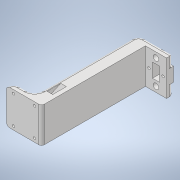
# Autodesk Inventor part: Joint_Tubes_1_2
Saved by Autodesk Inventor 2022.3 (Build 263350000, 350)
## iProperties
Created: 2023-03-29
Part Number: Joint_Tubes_1_2
Material: Generic
Document SubType Name: Modeling
Designer: Manuel Hueso Béjar
Density: 1 g/cm^3
Appearance: Default
Author: Manuel Hueso Béjar
Autodesk Inventor part; units mm, degrees
ref_plane "YZ Plane" through (0, 0, 0) normal (1, 0, 0) x (0, 1, 0)
ref_plane "XZ Plane" through (0, 0, 0) normal (0, 1, 0) x (-1, 0, 0)
ref_plane "XY Plane" through (0, 0, 0) normal (0, 0, 1) x (1, 0, 0)
sketch "Sketch1" plane through (0, 0, 0) normal (0, 1, 0) x (-1, 0, 0)
  line L0 (-10, 74) -> (10, 74)
  line L1 (10, 74) -> (10, -74)
  line L2 (10, -74) -> (-10, -74)
  line L3 (-10, -74) -> (-10, 74)
  line L4 (-10, 74) -> (10, -74) construction
  line L5 (10, 74) -> (-10, -74) construction
  line L6 (-10, 74) -> (40, 74)
  line L7 (40, 74) -> (40, 64)
  line L8 (40, 64) -> (-10, 64)
  line L9 (-10, 64) -> (-10, 74)
  line L10 (10, -74) -> (-40, -74)
  line L11 (-40, -74) -> (-40, -84)
  line L12 (-40, -84) -> (10, -84)
  line L13 (10, -84) -> (10, -74)
  point P0 (0, 0)
  point P1 (-10, -74)
  point P2 (10, 64)
  dimension "d0" = 20
  dimension "d1" = 148
  dimension "d2" = 50
  dimension "d3" = 10
  dimension "d4" = 50
  dimension "d5" = 10
  constraints: 28 end point, 6 parallel, 3 horizontal, 3 perpendicular, 2 midpoint
  measures "d0" distance of L1.end L2.end
  measures "d1" distance of L0.end L1.end
  measures "d2" distance of L7.end L8.end
  measures "d3" distance of L6.end L7.end
  measures "d4" distance of L12.end L11.end
  measures "d5" distance of L11.end L10.end
extrude "Extrusion1" add sketch "Sketch1" along normal blind 50
fillet "Fillet1" radius 10 2 edges at (-10, 25, -84) (-10, 25, 64)
fillet "Fillet2" radius 5 14 edges at (19.9999, 50, -84) (-10, 50, -9.9999) (-10, 50, -74) (-12.9289, 50, 61.0711) (-29.9999, 50, 64) (-7.0711, 50, -81.0711) (-10, 0, -74) (-7.0711, 0, -81.0711) (-10, 0, -9.9999) (-12.9289, 0, 61.0711) (-29.9999, 0, 64) (19.9999, 0, -84) (-40, 50, 69) (-40, 0, 69)
fillet "Fillet3" radius 10 3 edges at (-38.5355, 48.5355, 65.4645) (-38.5355, 1.4645, 65.4645) (-40, 25, 64)
sketch "Sketch2" plane through (10, 0, 74) normal (0, 0, 1) x (1, 0, 0)
  line L0 (0, 50) -> (-10, 50)
  line L1 (-10, 50) -> (-10, 45)
  line L2 (-10, 45) -> (0, 45)
  line L3 (0, 45) -> (0, 50)
  line L4 (-10, 0) -> (-10, 5) projected
  line L5 (0, 0) -> (-10, 0)
  line L6 (-10, 0) -> (-10, 5)
  line L7 (-10, 5) -> (0, 5)
  line L8 (0, 5) -> (0, 0)
  line L9 (0, 50) -> (-40, 50)
  line L10 (-40, 50) -> (-40, 45)
  line L11 (-40, 45) -> (0, 45)
  line L12 (0, 45) -> (0, 50)
  line L13 (0, 0) -> (-40, 0)
  line L14 (-40, 0) -> (-40, 5)
  line L15 (-40, 5) -> (0, 5)
  line L16 (0, 5) -> (0, 0)
  circle A0 centre (-10, 5) radius 1.7
  circle A1 centre (-10, 45) radius 1.7
  circle A2 centre (-40, 5) radius 1.7
  circle A3 centre (-40, 45) radius 1.7
  dimension "d11" = 10
  dimension "d12" = 5
  dimension "d13" = 10
  dimension "d14" = 5
  dimension "d15" = 40
  dimension "d16" = 5
  dimension "d17" = 40
  dimension "d18" = 5
  dimension "d19" = 3.4
  dimension "d20" = 3.4
  dimension "d21" = 3.4
  dimension "d22" = 3.4
  constraints: 32 end point, 8 parallel, 4 centre point, 4 coincident, 4 horizontal, 4 perpendicular
  measures "d11" distance of L2.end L1.end
  measures "d12" distance of L1.end L0.end
  measures "d13" distance of L4.end L7.end
  measures "d14" distance of L5.end L4.end
  measures "d15" distance of L11.end L10.end
  measures "d16" distance of L10.end L9.end
  measures "d17" distance of L14.end L15.end
  measures "d18" distance of L13.end L14.end
  measures "d19" diameter of A0
  measures "d20" diameter of A1
  measures "d21" diameter of A2
  measures "d22" diameter of A3
extrude "Extrusion2" cut sketch "Sketch2" against normal up to surface (10 mm away) contours A1 L2 L1 | L1 L11 A1 | A1 L11 L2 | A3 L11 L10 | L10 L11 A3 | A0 L15 L4 | L4 L7 A0 | L15 A0 L7 | A2 L15 L14 | L14 L15 A2
sketch "Sketch3" plane through (-20, 5, 64) normal (0, 0, -1) x (-1, 0, 0)
  circle A0 centre (10, 40) radius 1.7 projected
  arc A1 (10, 1.7) -> (8.3, 0) centre (10, 0) ccw projected
  line L0 (10, 40) -> (10, 0)
  point P0 (-20, -5)
  constraints: 2 end point, 1 vertical
hole "Hole1" at (-30, 45, 64) at (-30, 5, 64) direction (0, 0, 1) diameter 3.4 depth 2.2 countersink diameter 6 countersink angle 90
sketch "Sketch4" plane through (0, 45, 64) normal (0, 0, 1) x (1, 0, 0)
  line L0 (-4, -4) -> (4, -4)
  line L1 (4, -4) -> (4, 4)
  line L2 (4, 4) -> (-4, 4)
  line L3 (-4, 4) -> (-4, -4)
  line L4 (40, 0) -> (0, 0) projected
  line L5 (-4, -4) -> (4, 4) construction
  line L6 (4, -4) -> (-4, 4) construction
  point P0 (0, -45)
  dimension "d32" = 8
  dimension "d33" = 8
  constraints: 12 end point, 2 midpoint, 2 parallel, 1 horizontal, 1 perpendicular
  measures "d32" distance of L2.end L1.end
  measures "d33" distance of L1.end L0.end
sketch "Sketch5" plane through (10, 0, 74) normal (1, 0, 0) x (0, 0, -1)
  line L0 (0, 45) -> (20, 45)
  line L1 (20, 45) -> (20, 50)
  line L2 (20, 50) -> (0, 50)
  line L3 (0, 50) -> (0, 45)
  line L4 (20, 47.5) -> (40, 47.5)
  line L5 (40, 47.5) -> (40, 56.5)
  line L6 (40, 56.5) -> (20, 56.5)
  line L7 (20, 56.5) -> (20, 47.5)
  line L8 (20, 47.5) -> (40, 56.5)
  line L9 (0, 50) -> (148, 50) projected
  line L10 (0, 0) -> (0, 50) projected
  line L11 (20, 47.5) -> (10, 47.5)
  point P0 (74, 0)
  point P1 (148, 50)
  dimension "d34" = 20
  dimension "d35" = 5
  dimension "d36" = 20
  dimension "d37" = 9
  dimension "d38" = 0
  dimension "d39" = 0
  constraints: 20 end point, 4 parallel, 3 horizontal, 2 perpendicular, 1 midpoint, 1 other
  measures "d34" distance of L2.end L1.end
  measures "d35" distance of L1.end L0.end
  measures "d36" distance of L6.end L5.end
  measures "d37" distance of L5.end L4.end
  measures "d38" vertical extent of L2
  measures "d39" distance between parallel lines of L10 L3
sweep "Sweep1" cut profiles "Sketch4" path "Sketch5" path curves L11 L8
sketch "Sketch6" plane through (0, 5, 64) normal (0, 0, 1) x (1, 0, 0)
  line L0 (-4, -4) -> (4, -4)
  line L1 (4, -4) -> (4, 4)
  line L2 (4, 4) -> (-4, 4)
  line L3 (-4, 4) -> (-4, -4)
  line L4 (-10, 0) -> (0, 0) projected
  line L5 (-4, -4) -> (4, 4) construction
  line L6 (4, -4) -> (-4, 4) construction
  point P0 (0, -5)
  dimension "d42" = 8
  dimension "d43" = 8
  constraints: 12 end point, 2 midpoint, 2 parallel, 1 horizontal, 1 perpendicular
  measures "d42" distance of L2.end L1.end
  measures "d43" distance of L1.end L0.end
sketch "Sketch7" plane through (10, 0, 74) normal (1, 0, 0) x (0, 0, -1)
  line L0 (5, 0) -> (0, 0) projected
  line L1 (0, 0) -> (20, 0)
  line L2 (20, 0) -> (20, 5)
  line L3 (20, 5) -> (0, 5)
  line L4 (0, 5) -> (0, 0)
  line L5 (20, 2.5) -> (10, 2.5)
  line L6 (20, 2.5) -> (40, 2.5)
  line L7 (40, 2.5) -> (40, -6.5)
  line L8 (40, -6.5) -> (20, -6.5)
  line L9 (20, -6.5) -> (20, 2.5)
  line L10 (20, 2.5) -> (40, -6.5)
  point P0 (74, 0)
  dimension "d44" = 20
  dimension "d45" = 5
  dimension "d46" = 20
  dimension "d47" = 9
  constraints: 20 end point, 4 parallel, 3 horizontal, 2 perpendicular, 1 midpoint
  measures "d44" distance of L3.end L2.end
  measures "d45" distance of L2.end L1.end
  measures "d46" distance of L7.end L8.end
  measures "d47" distance of L6.end L7.end
sweep "Sweep2" cut profiles "Sketch6" path "Sketch7" path curves L5 L10
sketch "Sketch8" plane through (10, 0, -74) normal (0, 0, 1) x (1, 0, 0)
  line L0 (0, 50) -> (30, 50) projected
  line L1 (0, 0) -> (0, 50) projected
  line L2 (30, 50) -> (0, 50)
  line L3 (0, 50) -> (0, 0)
  line L4 (0, 0) -> (30, 0)
  line L5 (30, 0) -> (30, 50)
  line L6 (15, 50) -> (15, 0)
  line L7 (20, 15) -> (10, 15)
  line L8 (10, 15) -> (10, 35)
  line L9 (10, 35) -> (20, 35)
  line L10 (20, 35) -> (20, 15)
  line L11 (20, 15) -> (10, 35) construction
  line L12 (10, 15) -> (20, 35) construction
  line L13 (15, 50) -> (15, 35)
  line L14 (15, 0) -> (15, 15)
  circle A0 centre (15, 42.5) radius 4
  circle A1 centre (15, 7.5) radius 4
  point P0 (-10, 0)
  point P1 (15, 25)
  dimension "d50" = 10
  dimension "d51" = 20
  dimension "d52" = 8
  dimension "d53" = 8
  constraints: 26 end point, 9 midpoint, 4 parallel, 2 centre point, 2 horizontal, 2 perpendicular
  measures "d50" distance of L8.end L9.end
  measures "d51" distance of L7.end L8.end
  measures "d52" diameter of A0
  measures "d53" diameter of A1
extrude "Extrusion3" cut sketch "Sketch8" against normal through all contours A0 L6 | L6 A0 | A1 L6 | L6 A1
extrude "Extrusion4" cut sketch "Sketch8" against normal through all contours L9 L10 L7 L6 | L6 L7 L8 L9
sketch "Sketch9" plane through (0, 5, -84) normal (0, 0, -1) x (-1, 0, 0)
  circle A0 centre (-25, 2.5) radius 4 projected
  circle A1 centre (-25, 2.5) radius 6
  arc A2 (-28.1225, 40) -> (-21.8775, 40) centre (-25, 37.5) ccw projected
  circle A3 centre (-25, 37.5) radius 6
  point P0 (0, -5)
  dimension "d58" = 12
  dimension "d59" = 12
  constraints: 2 centre point, 2 coincident
  measures "d58" diameter of A1
  measures "d59" diameter of A3
extrude "Extrusion5" cut sketch "Sketch9" against normal blind 2 contours A0 | A1 | A3
fillet "Fillet5" radius 4 1 edges at (10, 25, 74)
sketch "Sketch12" plane through (-10, 5, 54) normal (-1, 0, 0) x (0, 0, 1)
  line L0 (-128, 40) -> (0, 40) construction
  line L1 (0, 40) -> (0, 0) construction
  line L2 (0, 0) -> (-128, 0) construction
  line L3 (-128, 0) -> (-128, 40) construction
  line L4 (-128, 40) -> (0, 40) projected
  line L5 (-128, 0) -> (-128, 40) projected
  line L6 (-118.4814, 5) -> (-108.3679, 35)
  line L7 (-108.3679, 35) -> (-103.4571, 35)
  line L8 (-103.4571, 35) -> (-93.3436, 5)
  line L9 (-93.3436, 5) -> (-97.5494, 5)
  line L10 (-97.5494, 5) -> (-100.2723, 13.3874)
  line L11 (-100.2723, 13.3874) -> (-111.7229, 13.3874)
  line L12 (-111.7229, 13.3874) -> (-114.4457, 5)
  line L13 (-114.4457, 5) -> (-118.4814, 5)
  line L14 (-101.3663, 16.7909) -> (-106.0097, 30.9157)
  line L15 (-106.0097, 30.9157) -> (-110.6289, 16.7909)
  line L16 (-110.6289, 16.7909) -> (-101.3663, 16.7909)
  line L17 (-73.1167, 5) -> (-90.4992, 5)
  line L18 (-90.4992, 5) -> (-90.4992, 35)
  line L19 (-90.4992, 35) -> (-86.5122, 35)
  line L20 (-86.5122, 35) -> (-86.5122, 8.5494)
  line L21 (-86.5122, 8.5494) -> (-73.1167, 8.5494)
  line L22 (-73.1167, 8.5494) -> (-73.1167, 5)
  line L23 (-59.5267, 5) -> (-71.1475, 5)
  line L24 (-71.1475, 5) -> (-71.1475, 8.0632)
  line L25 (-71.1475, 8.0632) -> (-67.3306, 8.0632)
  line L26 (-67.3306, 8.0632) -> (-67.3306, 31.9368)
  line L27 (-67.3306, 31.9368) -> (-71.1475, 31.9368)
  line L28 (-71.1475, 31.9368) -> (-71.1475, 35)
  line L29 (-71.1475, 35) -> (-59.5267, 35)
  line L30 (-59.5267, 35) -> (-59.5267, 31.9368)
  line L31 (-59.5267, 31.9368) -> (-63.3436, 31.9368)
  line L32 (-63.3436, 31.9368) -> (-63.3436, 8.0632)
  line L33 (-63.3436, 8.0632) -> (-59.5267, 8.0632)
  line L34 (-59.5267, 8.0632) -> (-59.5267, 5)
  spline S0 degree 2 poles (-42.8736, 4.4652) (-45.7909, 4.4652) (-50.7261, 6.4344) (-52.5251, 8.4036) knots 0 0 0 1 2 2 2
  spline S1 degree 2 poles (-52.5251, 8.4036) (-54.3242, 10.3485) (-56.2934, 16.1831) (-56.2934, 19.9757) knots 0 0 0 1 2 2 2
  spline S2 degree 2 poles (-56.2934, 19.9757) (-56.2934, 23.7439) (-54.3728, 29.3355) (-52.5494, 31.4019) knots 0 0 0 1 2 2 2
  spline S3 degree 2 poles (-52.5494, 31.4019) (-50.7504, 33.4198) (-45.8395, 35.5348) (-42.8007, 35.5348) knots 0 0 0 1 2 2 2
  spline S4 degree 2 poles (-42.8007, 35.5348) (-41.2934, 35.5348) (-38.6434, 35.0972) (-37.5251, 34.7569) knots 0 0 0 1 2 2 2
  spline S5 degree 2 poles (-37.5251, 34.7569) (-36.5527, 34.4408) (-34.5348, 33.5413) (-33.5381, 33.0065) knots 0 0 0 1 2 2 2
  line L35 (-33.5381, 33.0065) -> (-33.5381, 28.1929)
  line L36 (-33.5381, 28.1929) -> (-33.8541, 28.1929)
  spline S6 degree 2 poles (-33.8541, 28.1929) (-34.389, 28.6791) (-36.0421, 30.0405) (-37.2334, 30.6969) knots 0 0 0 1 2 2 2
  spline S7 degree 2 poles (-37.2334, 30.6969) (-38.376, 31.329) (-41.0746, 32.1313) (-42.825, 32.1313) knots 0 0 0 1 2 2 2
  spline S8 degree 2 poles (-42.825, 32.1313) (-44.7455, 32.1313) (-48.1734, 30.5511) (-49.4619, 29.0438) knots 0 0 0 1 2 2 2
  spline S9 degree 2 poles (-49.4619, 29.0438) (-50.7261, 27.5122) (-52.1361, 22.8687) (-52.1361, 19.9757) knots 0 0 0 1 2 2 2
  spline S10 degree 2 poles (-52.1361, 19.9757) (-52.1361, 16.8882) (-50.6532, 12.4392) (-49.3647, 10.9076) knots 0 0 0 1 2 2 2
  spline S11 degree 2 poles (-49.3647, 10.9076) (-48.1005, 9.4246) (-44.7212, 7.9173) (-42.825, 7.9173) knots 0 0 0 1 2 2 2
  spline S12 degree 2 poles (-42.825, 7.9173) (-41.0989, 7.9173) (-38.1572, 8.7682) (-37.0146, 9.4003) knots 0 0 0 1 2 2 2
  spline S13 degree 2 poles (-37.0146, 9.4003) (-35.9206, 10.0324) (-34.2917, 11.3452) (-33.8298, 11.8071) knots 0 0 0 1 2 2 2
  line L37 (-33.8298, 11.8071) -> (-33.5381, 11.8071)
  line L38 (-33.5381, 11.8071) -> (-33.5381, 7.0421)
  spline S14 degree 2 poles (-33.5381, 7.0421) (-34.5348, 6.5802) (-36.2853, 5.7293) (-37.5251, 5.3404) knots 0 0 0 1 2 2 2
  spline S15 degree 2 poles (-37.5251, 5.3404) (-38.8379, 4.9028) (-41.0746, 4.4652) (-42.8736, 4.4652) knots 0 0 0 1 2 2 2
  line L39 (-29.8185, 5) -> (-29.8185, 35)
  line L40 (-29.8185, 35) -> (-11.0502, 35)
  line L41 (-11.0502, 35) -> (-11.0502, 31.4506)
  line L42 (-11.0502, 31.4506) -> (-25.8314, 31.4506)
  line L43 (-25.8314, 31.4506) -> (-25.8314, 23.2334)
  line L44 (-25.8314, 23.2334) -> (-12.047, 23.2334)
  line L45 (-12.047, 23.2334) -> (-12.047, 19.684)
  line L46 (-12.047, 19.684) -> (-25.8314, 19.684)
  line L47 (-25.8314, 19.684) -> (-25.8314, 8.5494)
  line L48 (-25.8314, 8.5494) -> (-11.0502, 8.5494)
  line L49 (-11.0502, 8.5494) -> (-11.0502, 5)
  line L50 (-11.0502, 5) -> (-29.8185, 5)
  point P0 (-54, -5)
  dimension "d78" = 128
  dimension "d79" = 40
  dimension "d80" = 0
  dimension "d81" = 0
  constraints: 2 other
  measures "d78" distance of L0.start L0.end
  measures "d79" distance of L2.end L0.start
  measures "d80" distance between parallel lines of L4 L0
  measures "d81" distance between parallel lines of L5 L3
emboss "Emboss1" sketch "Sketch12" operation cut depth 1 direction (1, 0, 0)
sketch "Sketch13" plane through (0, 5, -84) normal (0, 0, -1) x (-1, 0, 0)
  line L0 (-20, 10) -> (-20, 30) projected
  line L1 (-20, 20) -> (-15, 20)
  line L2 (-30, 30) -> (-30, 10) projected
  line L3 (-30, 20) -> (-35, 20)
  point P0 (0, -5)
  dimension "d85" = 5
  dimension "d86" = 5
  constraints: 4 end point, 2 horizontal, 2 midpoint
  measures "d85" distance of L1.start L1.end
  measures "d86" distance of L3.start L3.end
hole "Hole4" at (35, 25, -84) at (15, 25, -84) direction (0, 0, 1) diameter 3.4 end through all counterbore diameter 4.1 counterbore depth 5.1
sketch "Sketch14" plane through (0, 50, 0) normal (0, 1, 0) x (1, 0, 0)
  line L0 (40, 84) -> (40, 79) projected
  line L1 (40, 84) -> (34, 84)
  line L2 (34, 84) -> (34, 78)
  line L3 (34, 78) -> (40, 78)
  line L4 (40, 78) -> (40, 84)
  circle A0 centre (34, 78) radius 6
  point P0 (0, 0)
  dimension "d94" = 6
  dimension "d95" = 6
  constraints: 8 end point, 2 parallel, 1 coincident, 1 horizontal, 1 perpendicular, 3 other
  measures "d94" distance of L3.end L2.end
  measures "d95" distance of L2.end L1.end
extrude "Extrusion6" cut sketch "Sketch14" against normal blind 15 contours L0 L4 A0 L1
sketch "Sketch15" plane through (0, 0, 0) normal (0, -1, 0) x (1, 0, 0)
  line L0 (40, -84) -> (40, -78) projected
  line L1 (40, -84) -> (34, -84)
  line L2 (34, -84) -> (34, -78)
  line L3 (34, -78) -> (40, -78)
  line L4 (40, -78) -> (40, -84)
  circle A0 centre (34, -78) radius 6
  point P0 (0, 0)
  dimension "d98" = 6
  dimension "d99" = 6
  constraints: 8 end point, 2 parallel, 1 coincident, 1 horizontal, 1 perpendicular, 3 other
  measures "d98" distance of L2.end L3.end
  measures "d99" distance of L1.end L2.end
extrude "Extrusion7" cut sketch "Sketch15" against normal blind 15 contours L1 A0 L0
body "Solid1"
